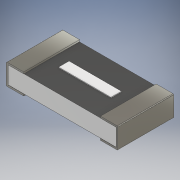
# Autodesk Inventor part: 21-1001
Saved by Autodesk Inventor 2018 (Build 220112000, 112)
## iProperties
Created: 2019-09-21
Part Number: 21-1001
Material: Copper
Document SubType Name: Modeling
Designer: Bradley
Density: 8.94 g/cm^3
Appearance: Smooth - White
Author: Bradley
Autodesk Inventor part; units mm, degrees
ref_plane "YZ Plane" through (0, 0, 0) normal (1, 0, 0) x (0, 1, 0)
ref_plane "XZ Plane" through (0, 0, 0) normal (0, 1, 0) x (-1, 0, 0)
ref_plane "XY Plane" through (0, 0, 0) normal (0, 0, 1) x (1, 0, 0)
sketch "Sketch1" plane through (0, 0, 0) normal (0, 1, 0) x (-1, 0, 0)
  line L0 (1.55, 0.25) -> (-1.55, 0.25)
  line L1 (-1.55, 0.25) -> (-1.55, -0.25)
  line L2 (-1.55, -0.25) -> (1.55, -0.25)
  line L3 (1.55, -0.25) -> (1.55, 0.25)
  line L4 (1.1, 0.25) -> (1.1, 0.3)
  line L5 (1.1, 0.3) -> (1.6, 0.3)
  line L6 (1.6, 0.3) -> (1.6, -0.3)
  line L7 (1.6, -0.3) -> (1.1, -0.3)
  line L8 (1.1, -0.3) -> (1.1, -0.25)
  line L9 (-1.1, 0.25) -> (-1.1, 0.3)
  line L10 (-1.1, 0.3) -> (-1.6, 0.3)
  line L11 (-1.6, 0.3) -> (-1.6, -0.3)
  line L12 (-1.6, -0.3) -> (-1.1, -0.3)
  line L13 (-1.1, -0.25) -> (-1.1, -0.3)
  line L14 (1.1, 0.25) -> (-1.1, 0.25)
  point P0 (0, 0)
  point P1 (0, 0.25)
  point P2 (1.55, 0)
  dimension "d0" = 3.2
  dimension "d1" = 0.05
  dimension "d2" = 0.05
  dimension "d3" = 0.6
  dimension "d4" = 0.5
  constraints: 30 end point, 12 point on line, 7 perpendicular, 3 collinear, 3 midpoint, 2 parallel, 1 horizontal, 1 horizontal alignment, 1 vertical, 1 vertical alignment
  measures "d0" distance between parallel lines of L11 L6
  measures "d1" distance of L7.end L8.end
  measures "d2" distance between parallel lines of L6 L3
  measures "d3" distance of L5.end L6.end
  measures "d4" distance of L6.end L7.end
extrude "Extrusion1" add sketch "Sketch1" along normal mid plane 1.6 contours L0 L4 L5 L6 L7 L8 L2 L3 | L0 L1 L2 L13 L12 L11 L10 L9
extrude "Extrusion2" add sketch "Sketch1" along normal mid plane 1.59 contours L3 L2 L1 L0
sketch "Sketch2" plane through (-1.1, -0.795, 0.25) normal (0, 0, 1) x (1, 0, 0)
  line L0 (0, 0) -> (0, 1.59) projected
  line L1 (2.2, 0) -> (0, 0) projected
  line L2 (2.2, 0) -> (2.2, 1.59) projected
  line L3 (0, 1.59) -> (2.2, 1.59) projected
  line L4 (0, 0.795) -> (2.2, 0.795) construction
  line L5 (1.85, 0.645) -> (0.35, 0.645)
  line L6 (0.35, 0.645) -> (0.35, 0.945)
  line L7 (0.35, 0.945) -> (1.85, 0.945)
  line L8 (1.85, 0.945) -> (1.85, 0.645)
  line L9 (1.85, 0.645) -> (0.35, 0.945) construction
  line L10 (0.35, 0.645) -> (1.85, 0.945) construction
  point P0 (1.1, 0.795)
  dimension "d12" = 1.5
  dimension "d13" = 0.3
  constraints: 14 end point, 4 midpoint, 2 parallel, 1 horizontal, 1 perpendicular
  measures "d12" distance of L6.end L7.end
  measures "d13" distance of L5.end L6.end
extrude "Extrusion3" add sketch "Sketch2" along normal blind 0.02 contours L5 L6 L7 L8
fillet "Fillet1" radius 0.02 4 edges at (-1.6, 0, 0.3) (-1.6, 0, -0.3) (1.6, 0, 0.3) (1.6, 0, -0.3)
equation "\"d2\" = d1"
body "Solid1"
